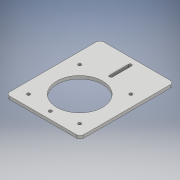
# Autodesk Inventor part: Адаптер для считывателя Bolid Proxy-2MA часть 1
Saved by Autodesk Inventor 2018 (Build 220112000, 112)
## iProperties
Created: 2019-06-30
Part Number: Адаптер для считывателя Bolid Proxy-2MA часть 1
Material: Типовые
Document SubType Name: Modeling
Designer: KV33_HP1
Density: 1 g/cm^3
Appearance: По умолчанию
Author: KV33_HP1
Autodesk Inventor part; units mm, degrees
ref_plane "YZ Plane" through (0, 0, 0) normal (1, 0, 0) x (0, 1, 0)
ref_plane "XZ Plane" through (0, 0, 0) normal (0, 1, 0) x (-1, 0, 0)
ref_plane "XY Plane" through (0, 0, 0) normal (0, 0, 1) x (1, 0, 0)
sketch "Эскиз1" plane through (0, 0, 0) normal (0, 0, 1) x (1, 0, 0)
  line L0 (5, 0) -> (92, 0)
  line L1 (97, 5) -> (97, 118)
  line L2 (92, 123) -> (5, 123)
  line L3 (0, 118) -> (0, 5)
  circle A0 centre (48.5, 48) radius 30
  circle A1 centre (15, 81.5) radius 2
  circle A2 centre (82, 81.5) radius 2
  circle A3 centre (82, 14.5) radius 2
  circle A4 centre (15, 14.5) radius 2
  arc A5 (5, 123) -> (0, 118) centre (5, 118) ccw
  arc A6 (97, 118) -> (92, 123) centre (92, 118) ccw
  arc A7 (92, 0) -> (97, 5) centre (92, 5) ccw
  arc A8 (0, 5) -> (5, 0) centre (5, 5) ccw
  circle A9 centre (48.5, 9.5) radius 2
  arc A10 (46.5, 89) -> (50.5, 89) centre (48.5, 89) ccw
  arc A11 (50.5, 114) -> (46.5, 114) centre (48.5, 114) ccw
  line L4 (46.5, 89) -> (46.5, 114)
  line L5 (50.5, 114) -> (50.5, 89)
  point P0 (0, 0)
  point P1 (97, 123)
  point P2 (0, 123)
  dimension "d7" = 4
  dimension "d8" = 4
  dimension "d9" = 4
  dimension "d10" = 5
  dimension "d21" = 4
  dimension "d22" = 4
  dimension "d23" = 4
  constraints: 12 centre point, 12 end point, 12 point on circle, 10 tangent, 6 point on line, 3 equal radius, 3 parallel, 1 horizontal, 1 perpendicular, 1 vertical
  measures "d7" diameter of A1
  measures "d8" diameter of A3
  measures "d9" diameter of A4
  measures "d10" radius of A5
  measures "d21" diameter of A9
  measures "d22" diameter of A10
  measures "d23" diameter of A11
extrude "Выдавливание1" add sketch "Эскиз1" along normal blind 4
